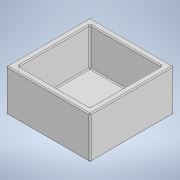
# Autodesk Inventor part: S-12685 Insulated Box
Saved by Autodesk Inventor 2022 (Build 260153000, 153)
## iProperties
Created: 2022-01-24
Part Number: S-12685 Insulated Box
Material: Generic
Document SubType Name: Modeling
Designer: Caleb
Density: 1 g/cm^3
Appearance: Default
Author: Caleb
Autodesk Inventor part; units mm, degrees
ref_plane "YZ Plane" through (0, 0, 0) normal (1, 0, 0) x (0, 1, 0)
ref_plane "XZ Plane" through (0, 0, 0) normal (0, 1, 0) x (-1, 0, 0)
ref_plane "XY Plane" through (0, 0, 0) normal (0, 0, 1) x (1, 0, 0)
sketch "Sketch1" plane through (0, 0, 0) normal (0, 1, 0) x (-1, 0, 0)
  line L0 (-215.9, -215.9) -> (215.9, -215.9)
  line L1 (215.9, -215.9) -> (215.9, 215.9)
  line L2 (215.9, 215.9) -> (-215.9, 215.9)
  line L3 (-215.9, 215.9) -> (-215.9, -215.9)
  line L4 (-215.9, -215.9) -> (215.9, 215.9) construction
  line L5 (215.9, -215.9) -> (-215.9, 215.9) construction
  line L6 (-254, 254) -> (254, 254)
  line L7 (254, 254) -> (254, -254)
  line L8 (254, -254) -> (-254, -254)
  line L9 (-254, -254) -> (-254, 254)
  line L10 (-254, 254) -> (254, -254) construction
  line L11 (254, 254) -> (-254, -254) construction
  point P0 (0, 0)
  dimension "d0" = 431.8
  dimension "d1" = 431.8
  dimension "d2" = 508
  dimension "d3" = 508
  constraints: 24 end point, 4 midpoint, 4 parallel, 2 horizontal, 2 perpendicular
  measures "d0" distance of L2.end L1.end
  measures "d1" distance of L1.end L0.end
  measures "d2" distance of L7.end L8.end
  measures "d3" distance of L6.end L7.end
extrude "Extrusion1" add sketch "Sketch1" along normal blind 228.6
sketch "Sketch2" plane through (0, 0, 0) normal (0, -1, 0) x (1, 0, 0)
  line L0 (-254, 254) -> (254, 254) projected
  line L1 (254, 254) -> (254, -254) projected
  line L2 (254, -254) -> (-254, -254) projected
  line L3 (-254, -254) -> (-254, 254) projected
  point P0 (0, 0)
extrude "Extrusion2" add sketch "Sketch2" along normal blind 25.4
fillet "Fillet1" radius 6.35 24 edges at (254, 101.6, -254) (0, 228.6, -254) (254, 228.6, 0) (254, 101.6, 254) (254, -25.4, 0) (0, -25.4, -254) (0, 228.6, -215.9) (-215.9, 228.6, 0) (-215.9, 0, 0) (0, 0, 215.9) (-215.9, 114.3, 215.9) (0, 228.6, 215.9) (0, 228.6, 254) (-254, 228.6, 0) (215.9, 228.6, 0) (215.9, 0, 0) (0, 0, -215.9) (0, -25.4, 254) (-254, 101.6, 254) (-254, -25.4, 0) (-215.9, 114.3, -215.9) (215.9, 114.3, -215.9) (215.9, 114.3, 215.9) (-254, 101.6, -254)
body "Solid1"
